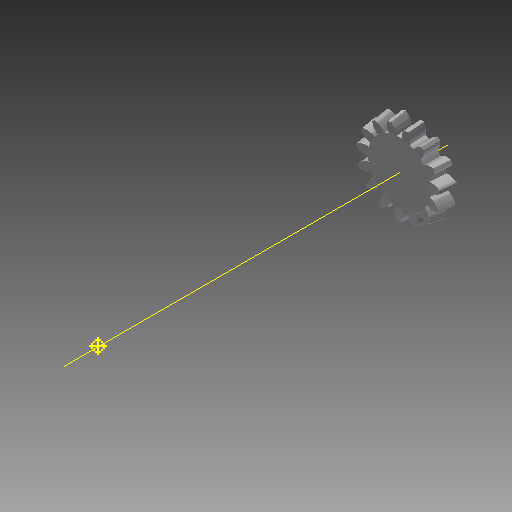
# Autodesk Inventor part: Bevel Gear2
Saved by Autodesk Inventor 2017 (Build 210142000, 142)
## iProperties
Created: 2017-01-10
Part Number: Bevel Gear2
Material: Steel, Mild
Document SubType Name: Modeling
Designer: David Kopala
Categories: <?xml version="1.0" encoding="UTF-16"?> <MemberInstance><Categories><FamilyTemplate><FamilyTemplateParameter ValueType="xs:double" Id="1" ObjectReferenceKey="da_z" ObjectType="kUserParameterObject"/><FamilyTemplateParameter ValueType="xs:double" Id="2" ObjectReferenceKey="da_b" ObjectType="kUserParameterObject"/><FamilyTemplateParameter ValueType="xs:double" Id="3" ObjectReferenceKey="da_beta" ObjectType="kUserParameterObject"/><FamilyTemplateParameter ValueType="xs:double" Id="4" ObjectReferenceKey="da_dae" ObjectType="kUserParameterObject"/><FamilyTemplateParameter ValueType="xs:double" Id="5" ObjectReferenceKey="da_ve" ObjectType="kUserParameterObject"/><FamilyTemplateParameter ValueType="xs:double" Id="6" ObjectReferenceKey="da_omega" ObjectType="kUserParameterObject"/><FamilyTemplateParameter ValueType="xs:string" Id="7" ObjectReferenceKey="EAIAABAAAAAAHwAAAAAAAIAAAAAAAAAA" ObjectType="83914240" SubObjectId="SurfaceGeometry"/></FamilyTemplate><ParamToTemplateMap><ParamToTemplate CategoryParameter="//CategoryParameter[@InternalName='046C89C9-8512-4d59-83FE-43B91F4F132A']" TemplateParameter="1"/><ParamToTemplate CategoryParameter="//CategoryParameter[@InternalName='2552DF32-E462-4b46-AEBF-C6C7768E72AC']" TemplateParameter="2"/><ParamToTemplate CategoryParameter="//CategoryParameter[@InternalName='C9EE641D-15FC-4fae-A226-E94C4372FDD7']" TemplateParameter="3"/><ParamToTemplate><ParamToTemplate CategoryParameter="//CategoryParameter[@InternalName='00B6519A-459B-49c7-AD84-2E56D39A5744']" ConstantValue="-0.000000"/></ParamToTemplate><ParamToTemplate><ParamToTemplate CategoryParameter="//CategoryParameter[@InternalName='04B31F0E-C7A6-4894-AA32-9629BEFACF47']" ConstantValue="1.000000"/></ParamToTemplate><ParamToTemplate><ParamToTemplate CategoryParameter="//CategoryParameter[@InternalName='43CBEC2E-7847-49e7-A936-2F7889FCB2D9']" ConstantValue="0.200000"/></ParamToTemplate><ParamToTemplate><ParamToTemplate CategoryParameter="//CategoryParameter[@InternalName='B1EFC894-105D-4ebd-86BF-FA20ED196853']" ConstantValue="0.300000"/></ParamToTemplate><ParamToTemplate><ParamToTemplate CategoryParameter="//CategoryParameter[@InternalName='51175063-3D10-4879-93E8-6246FE8B403D']" ConstantValue="2061532430.657340"/></ParamToTemplate><ParamToTemplate><ParamToTemplate CategoryParameter="//CategoryParameter[@InternalName='A3A52E27-4454-46a9-B0BD-C932399B70AF']" ConstantValue="0.300000"/></ParamToTemplate><ParamToTemplate CategoryParameter="//CategoryParameter[@InternalName='2A200944-5A8C-41ca-B96E-8520D2E510F1']" TemplateParameter="4"/><ParamToTemplate><ParamToTemplate CategoryParameter="//CategoryParameter[@InternalName='1A637F62-92C8-44bc-B81F-10802510B579']" ConstantValue="4.085515"/></ParamToTemplate><ParamToTemplate CategoryParameter="//CategoryParameter[@InternalName='B52DD4BE-6863-48fb-BF58-89EF6F9EC65C']" TemplateParameter="5"/><ParamToTemplate><ParamToTemplate CategoryParameter="//CategoryParameter[@InternalName='3956BFF2-84D2-457d-93C2-9B0613DEBA67']" ConstantValue="14.709325"/></ParamToTemplate><ParamToTemplate CategoryParameter="//CategoryParameter[@InternalName='739CFA02-461B-4bf8-8049-181FCAD8B28F']" TemplateParameter="6"/><ParamToTemplate><ParamToTemplate CategoryParameter="//CategoryParameter[@InternalName='A27E999F-E2CE-4481-8A2A-EBF499C4C3C5']" ConstantValue="-0.000000"/></ParamToTemplate><ParamToTemplate><ParamToTemplate CategoryParameter="//CategoryParameter[@InternalName='9E1B4470-B2D3-4ff1-B813-535BB4CDF51A']" ConstantValue="3523220.976809"/></ParamToTemplate><ParamToTemplate><ParamToTemplate CategoryParameter="//CategoryParameter[@InternalName='F8452263-BFF6-458c-9FB1-07C4B99E95CD']" ConstantValue="11397033.805607"/></ParamToTemplate><ParamToTemplate><ParamToTemplate CategoryParameter="//CategoryParameter[@InternalName='3E3BB259-FD49-497f-8171-6EBC954A3479']" ConstantValue="2.000000"/></ParamToTemplate><ParamToTemplate CategoryParameter="//CategoryParameter[@InternalName='27C3BAF2-7550-4e4b-AE2C-0DB134B7D9B7']" TemplateParameter="7"/></ParamToTemplateMap><Category DisplayName="Gear" InternalName="DC85795E-93AB-48d5-8EEE-5A27447B64BD" Mnemonic="Gear"><CategoryParameter DisplayName="z" InternalName="046C89C9-8512-4d59-83FE-43B91F4F132A" Mnemonic="z"/><CategoryParameter DisplayName="b" InternalName="2552DF32-E462-4b46-AEBF-C6C7768E72AC" Mnemonic="b"/><CategoryParameter DisplayName="||b|" InternalName="C9EE641D-15FC-4fae-A226-E94C4372FDD7" Mnemonic="beta"/><CategoryParameter DisplayName="x" InternalName="00B6519A-459B-49c7-AD84-2E56D39A5744" Mnemonic="x"/><CategoryParameter DisplayName="a*" InternalName="04B31F0E-C7A6-4894-AA32-9629BEFACF47" Mnemonic="a"/><CategoryParameter DisplayName="c*" InternalName="43CBEC2E-7847-49e7-A936-2F7889FCB2D9" Mnemonic="c"/><CategoryParameter DisplayName="r|.f|*" InternalName="B1EFC894-105D-4ebd-86BF-FA20ED196853" Mnemonic="rf"/><CategoryParameter DisplayName="E" InternalName="51175063-3D10-4879-93E8-6246FE8B403D" Mnemonic="E"/><CategoryParameter DisplayName="||m|" InternalName="A3A52E27-4454-46a9-B0BD-C932399B70AF" Mnemonic="mi"/><Category DisplayName="BevelGear" InternalName="0C98F69A-0C2B-4791-B2FE-7691BB227E77" Mnemonic="BevelGear"><CategoryParameter DisplayName="d|.ae|" InternalName="2A200944-5A8C-41ca-B96E-8520D2E510F1" Mnemonic="dae"/><CategoryParameter DisplayName="d|.ai|" InternalName="1A637F62-92C8-44bc-B81F-10802510B579" Mnemonic="dai"/><CategoryParameter DisplayName="A|.e|" InternalName="B52DD4BE-6863-48fb-BF58-89EF6F9EC65C" Mnemonic="ve"/><CategoryParameter DisplayName="A|.i|" InternalName="3956BFF2-84D2-457d-93C2-9B0613DEBA67" Mnemonic="vi"/><CategoryParameter DisplayName="||S|" InternalName="739CFA02-461B-4bf8-8049-181FCAD8B28F" Mnemonic="omega"/><CategoryParameter DisplayName="x|.t|" InternalName="A27E999F-E2CE-4481-8A2A-EBF499C4C3C5" Mnemonic="xt"/><CategoryParameter DisplayName="||s||.Flim|" InternalName="9E1B4470-B2D3-4ff1-B813-535BB4CDF51A" Mnemonic="sFlim"/><CategoryParameter DisplayName="||s||.Hlim|" InternalName="F8452263-BFF6-458c-9FB1-07C4B99E95CD" Mnemonic="sHlim"/><CategoryParameter DisplayName="type" InternalName="3E3BB259-FD49-497f-8171-6EBC954A3479" Mnemonic="type"/><CategoryParameter DisplayName="PitchDiameter" InternalName="27C3BAF2-7550-4e4b-AE2C-0DB134B7D9B7" Mnemonic="IDS_PITCHDIAM"/></Category></Category></Categories></MemberInstance>
Mass: 60.9118 g
Surface Area: 34.3074 cm^2
Volume: 7.7496 cm^3
Density: 7.86 g/cm^3
Appearance: Steel
CustomPartVersion: 1
Author: David Kopala
Autodesk Inventor part; units mm, degrees
ref_plane "XZ Plane" through (0, 0, 0) normal (0, 1, 0) x (-1, 0, 0)
ref_plane "Mesh Plane2" through (0, 0, 0) normal (0.9781476, 0.2079117, 0) x (0, 0, 1)
sketch "Teeth Body Sketch" plane through (0, 0, 0) normal (1, 0, 0) x (0, 1, 0)
  line L0 (0, 0) -> (16.0248, -155.312) construction
  line L1 (16.0248, -155.312) -> (21.4759, -154.6417)
  line L2 (21.4759, -154.6417) -> (0, 0) construction
  line L3 (19.05, -154.94) -> (0, 0) construction
  line L4 (15.2426, -147.7307) -> (20.4276, -147.0932)
  line L5 (16.0248, -155.312) -> (15.2426, -147.7307)
  line L6 (21.4759, -154.6417) -> (20.4276, -147.0932)
  line L7 (0, -187.8948) -> (0, 31.3158) projected
  line L8 (0, -154.94) -> (21.4759, -154.94) construction
  dimension "d0" = 38.1
  dimension "d1" = 32.0496
  dimension "d2" = 42.9517
  dimension "d3" = 7.62
  dimension "d4" = 154.6417
  constraints: 16 end point, 4 point on line, 3 perpendicular, 2 collinear, 1 horizontal alignment, 1 vertical alignment
  measures "d0" diameter of L3.start L7
  measures "d1" diameter of L0.end L7
  measures "d2" diameter of L1.end L7
  measures "d3" distance between parallel lines of L1 L4
  measures "d4" vertical distance of L1.end L0.start
revolve "Teeth Body" add sketch "Teeth Body Sketch" angle 360 about axis through (0, 0, 0) along (0, 0, 1)
ref_plane "Tooth Plane" through (0, 19.05, -154.94) normal (0, -0.1220319, 0.9925262) x (1, 0, 0)
sketch "Start Sketch" plane through (0, 19.05, -154.94) normal (0, -0.1220319, 0.9925262) x (1, 0, 0)
  line L0 (0, -23.8477) -> (0, 8.7484) projected
  arc A0 (-1.2152, -3.7071) -> (-5.7872, 3.3611) centre (-8.4638, -3.383) ccw
  arc A1 (5.7872, 3.3611) -> (1.2152, -3.7071) centre (8.4638, -3.383) ccw
  line L1 (-1.2152, -3.7071) -> (1.2152, -3.7071)
  arc A2 (5.7872, 3.3611) -> (-5.7872, 3.3611) centre (0, -19.1934) ccw
  dimension "d7" = 7.2558
  dimension "d8" = 8.4638
  dimension "d9" = 15.8105
  dimension "d57" = 23.2852
  dimension "d58" = 15.4864
  constraints: 6 point on circle, 3 centre point, 3 symmetric about line, 2 end point, 1 coincident, 1 perpendicular, 1 other
  measures "d7" radius of A0
  measures "d8" horizontal distance of point (0, -19.193) A0.centre
  measures "d9" vertical distance of point (0, -19.193) A0.centre
  measures "d57" radius of A2
  measures "d58" distance from line of A2.centre L1
sketch "End Sketch" plane through (0, 18.0866, -147.1044) normal (0, -0.1220319, 0.9925262) x (1, 0, 0)
  line L0 (0, -22.656) -> (0, 8.3375) projected
  arc A0 (-1.1549, -3.5041) -> (-5.5004, 3.2137) centre (-8.0442, -3.1961) ccw
  arc A1 (5.5004, 3.2137) -> (1.1549, -3.5041) centre (8.0442, -3.1961) ccw
  line L1 (-1.1549, -3.5041) -> (1.1549, -3.5041)
  arc A2 (5.5004, 3.2137) -> (-5.5004, 3.2137) centre (0, -18.2228) ccw
  dimension "d12" = 6.8961
  dimension "d15" = 8.0442
  dimension "d16" = 15.0267
  dimension "d59" = 22.1309
  dimension "d60" = 14.7187
  constraints: 6 point on circle, 3 centre point, 3 symmetric about line, 2 end point, 1 coincident, 1 other
  measures "d12" radius of A0
  measures "d15" horizontal distance of A0.centre point (0, -18.223)
  measures "d16" vertical distance of A0.centre point (0, -18.223)
  measures "d59" radius of A2
  measures "d60" distance from line of A2.centre L1
loft "Loft" cut profiles "Start Sketch", "End Sketch"
pattern_circular "Circular Pattern" count 15 over 360 about axis through (0, 0, 0) along (0, 0, 1) of "Loft"
ref_plane "End Plane" through (0, 18.0866, -147.1044) normal (0, -0.1220319, 0.9925262) x (1, 0, 0)
sketch3d "3D Sketch Right"
ref_plane "End Plane Right" through (-2.8224, 17.865, -147.1044) normal (0.0190427, -0.120537, 0.9925262) x (0.9877496, 0.1560471, 0)
sketch "End Sketch Right" plane through (-2.8224, 17.865, -147.1044) normal (0.0190427, -0.120537, 0.9925262) x (0.9877496, 0.1560471, 0)
  arc A0 (-1.1549, -3.5041) -> (-5.5004, 3.2137) centre (-8.0442, -3.1961) ccw
  line L0 (0, -26.1029) -> (0, 11.7844) projected
  arc A1 (5.5004, 3.2137) -> (1.1549, -3.5041) centre (8.0442, -3.1961) ccw
  line L1 (-1.1549, -3.5041) -> (1.1549, -3.5041)
  arc A2 (5.5004, 3.2137) -> (-5.5004, 3.2137) centre (0, -18.2228) ccw
  dimension "d70" = 8.0442
  dimension "d71" = 15.0267
  dimension "d72" = 6.8961
  dimension "d73" = 14.7187
  dimension "d74" = 22.1309
  constraints: 6 point on circle, 3 centre point, 3 symmetric about line, 2 end point, 1 coincident, 1 perpendicular, 1 other
  measures "d70" horizontal distance of A2.centre A0.centre
  measures "d71" vertical distance of point (0, -18.223) A0.centre
  measures "d72" radius of A0
  measures "d73" distance from line of point (0, -18.223) L1
  measures "d74" radius of A2
feature "Loft Right" [suppressed]
pattern_circular "Circular Pattern Right" [suppressed]
sketch3d "3D Sketch Left"
ref_plane "End Plane Left" through (2.8111, 17.865, -147.1004) normal (-0.0189675, -0.1205404, 0.9925272) x (0.9878451, -0.1554414, 0)
sketch "End Sketch Left" plane through (2.8111, 17.865, -147.1004) normal (-0.0189675, -0.1205404, 0.9925272) x (0.9878451, -0.1554414, 0)
  line L0 (0, -55.3968) -> (0, 21.063) projected
  arc A0 (-1.1549, -3.5029) -> (-5.5004, 3.215) centre (-8.0442, -3.1948) ccw
  arc A1 (5.5004, 3.215) -> (1.1549, -3.5029) centre (8.0442, -3.1948) ccw
  line L1 (-1.1549, -3.5029) -> (1.1549, -3.5029)
  ellipse E0 centre (0, -17.9488) end of major axis (20.4276, -17.9488) minor radius 20.2749 projected
  arc A2 (5.5004, 3.215) -> (-5.5004, 3.215) centre (0, -18.2216) ccw
  dimension "d56" = 20.2749
  dimension "d30" = 6.8961
  dimension "d31" = 8.0442
  dimension "d32" = 15.0267
  dimension "d61" = 22.1309
  dimension "d62" = 14.7187
  constraints: 6 point on circle, 3 centre point, 3 symmetric about line, 2 end point, 1 coincident, 2 other
  measures "d30" radius of A0
  measures "d31" horizontal distance of point (0, -18.222) A0.centre
  measures "d32" vertical distance of A0.centre point (0, -18.222)
  measures "d61" radius of A2
  measures "d62" distance from line of point (0, -18.222) L1
feature "Loft Left" [suppressed]
pattern_circular "Circular Pattern Left" [suppressed]
sketch "Body Sketch" plane through (0, 0, 0) normal (1, 0, 0) x (0, 1, 0)
  line L0 (0, -158.0953) -> (0, -147.4808) projected
  line L1 (16.0248, -155.312) -> (15.2426, -147.7307) projected
  line L2 (15.2426, -147.7307) -> (0, -147.7307)
  line L3 (16.0248, -155.312) -> (0, -155.312)
  constraints: 4 end point, 2 perpendicular, 2 point on line
revolve "Fix Body" add sketch "Body Sketch" angle 360 about axis through (0, 0, 0) along (0, 0, 1)
sketch "Sketch6" plane through (0, 0, 0) normal (1, 0, 0) x (0, 1, 0)
  line L0 (19.05, -154.94) -> (0, 0) projected
  line L1 (0, -187.452) -> (0, 31.242) projected
surface revolve "Pitch Diameter" sketch "Sketch6" angle 360 about axis through (0, 0, 0) along (0, 0, 1) shown no curves L0
equation "\"d0\" = da_de"
equation "\"d1\" = da_dfe"
equation "\"d2\" = da_dae"
equation "\"d3\" = da_b"
equation "\"d4\" = da_ve"
equation "\"d7\" = fd_rr"
equation "\"d8\" = fd_x"
equation "\"d9\" = fd_y"
equation "\"d57\" = 0.5 * fd_dva + 0.3 * da_he"
equation "\"d58\" = 0.5 * fd_dva - 1.12 * da_he"
equation "\"da_teethtype\" = 0"
equation "\"da_b\" = 7.62"
equation "\"da_de\" = 38.1"
equation "\"da_dae\" = 42.95174"
equation "\"da_dfe\" = 32.04956"
equation "\"da_le\" = 156.10671"
equation "\"da_omega\" = 90deg"
equation "\"da_beta\" = 0"
equation "\"da_delta\" = 7.009384deg"
equation "\"da_alpha\" = 20deg"
equation "\"da_he\" = 5.49214"
equation "\"da_ve\" = 154.64174"
equation "\"da_zv\" = 15.112952"
equation "\"fd_loft\" = da_b + 0.05 * da_he"
equation "\"fd_x\" = fd_x1 + fd_x2"
equation "\"fd_y\" = fd_y1 - fd_y2"
equation "\"fd_dd\" = fd_dva - 0.8 * da_he"
equation "\"da_dvw\" = 38.3869"
equation "\"d11\" = fd_loft"
equation "\"da_dm\" = 37.17012"
equation "\"da_x\" = 0"
equation "\"da_m\" = 2.54"
equation "\"d50\" = da_omega"
equation "\"fd_rr\" = 7.255814"
equation "\"fd_dva\" = 43.275173"
equation "\"fd_x1\" = 1.991321"
equation "\"fd_x2\" = 6.472437"
equation "\"fd_y1\" = 19.089869"
equation "\"fd_y2\" = 3.279388"
body "Solid1"
body "Srf1"
